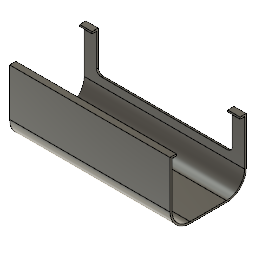
GT_motor_cover (Autodesk Fusion 360 design; units mm, degrees)
Autodesk Fusion 360 part; units mm, degrees
sketch "スケッチ1" plane through (0, 0, 0) normal (1, 0, 0) x (0, 1, 0)
  line L0 (-40, 36.5) -> (40, 36.5)
  line L1 (40, 36.5) -> (40, -13.5)
  line L2 (20, -33.5) -> (-20, -33.5)
  line L3 (-40, -13.5) -> (-40, 36.5)
  arc A0 (20, -33.5) -> (40, -13.5) centre (20, -13.5) ccw
  arc A1 (-40, -13.5) -> (-20, -33.5) centre (-20, -13.5) ccw
  line L4 (-42, 38.5) -> (42, 38.5)
  line L5 (42, 38.5) -> (42, -13.5)
  line L6 (20, -35.5) -> (-20, -35.5)
  line L7 (-42, -13.5) -> (-42, 38.5)
  arc A2 (20, -35.5) -> (42, -13.5) centre (20, -13.5) ccw
  arc A3 (-42, -13.5) -> (-20, -35.5) centre (-20, -13.5) ccw
  point P0 (-40, -33.5)
  dimension "d1" = 80
  dimension "d2" = 70
  dimension "d3" = 33.5
  dimension "d4" = 40
  dimension "d5" = 20
  dimension "d6" = 20
  dimension "d7" = 2
  dimension "d8" = 2
  dimension "d9" = 2
  dimension "d10" = 2
  dimension "d11" = 22
  dimension "d12" = 22
  constraint horizontal L0
  constraint vertical L1
  constraint horizontal L2
  constraint vertical L3
  constraint tangent L1 A0
  constraint tangent L2 A0
  constraint coincident P0 L2
  constraint coincident P0 L3
  constraint tangent L2 A1
  constraint tangent L3 A1
  constraint horizontal L4
  constraint vertical L5
  constraint horizontal L6
  constraint vertical L7
  constraint tangent L5 A2
  constraint tangent L6 A2
  constraint tangent L6 A3
  constraint tangent L7 A3
  measures "d1" distance of L0.start L0.end
  measures "d2" distance of L0.start P0
  measures "d3" distance of origin L2
  measures "d4" distance of origin L3
  measures "d5" radius of A0
  measures "d6" radius of A1
  measures "d7" distance of L1 L5
  measures "d8" distance of L0 L4
  measures "d9" distance of L3 L7
  measures "d10" distance of L2 L6
  measures "d11" radius of A2
  measures "d12" radius of A3
extrude "押し出し1" add sketch "スケッチ1" along normal mid plane 176.6
sketch "スケッチ2" plane through (0, 0, 0) normal (0, 0, 1) x (1, 0, 0)
  line L0 (-90, 35) -> (90, 35)
  line L1 (90, 35) -> (90, -35)
  line L2 (90, -35) -> (-90, -35)
  line L3 (-90, -35) -> (-90, 35)
  dimension "d15" = 180
  dimension "d16" = 90
  dimension "d17" = 70
  dimension "d18" = 35
  constraint horizontal L0
  constraint vertical L1
  constraint horizontal L2
  constraint vertical L3
  measures "d15" distance of L0.start L0.end
  measures "d16" distance of origin L3
  measures "d17" distance of L0.end L1.end
  measures "d18" distance of origin L0
extrude "押し出し2" cut sketch "スケッチ2" along normal blind 50
sketch "スケッチ3" plane through (0, 0, 0) normal (0, 1, 0) x (1, 0, 0)
  line L0 (74.5, -45.5) -> (-74.5, -45.5)
  line L1 (-74.5, -45.5) -> (-74.5, 4.5)
  line L2 (-74.5, 4.5) -> (74.5, 4.5)
  line L3 (74.5, 4.5) -> (74.5, -45.5)
  dimension "d21" = 149
  dimension "d22" = 74.5
  dimension "d23" = 50
  dimension "d29" = 4.5
  constraint horizontal L0
  constraint vertical L1
  constraint horizontal L2
  constraint vertical L3
  measures "d21" distance of L0.start L0.end
  measures "d22" distance of origin L1
  measures "d23" distance of L0.end L1.end
  measures "d29" distance of origin L2
extrude "押し出し3" cut sketch "スケッチ3" along normal blind 45
fillet "フィレット1" radius 5 2 edges at (74.5, 41, -4.5) (-74.5, 41, -4.5)
equation "d3 = ( 67 / 2 ) * 1 mm"
equation "d4 = ( 80 / 2 ) * 1 mm"
equation "d13 = ( 176.6 / 2 ) * 1 mm"
equation "d17 = 80 mm - 10 mm"
equation "d18 = ( 70 / 2 ) * 1 mm"
equation "d22 = ( 149 / 2 ) * 1 mm"
